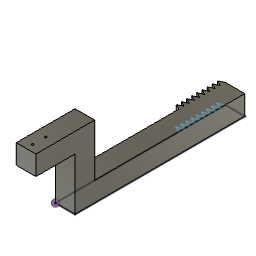
ClaspRight v1 (Autodesk Fusion 360 design; units mm, degrees)
Autodesk Fusion 360 part; units mm, degrees
sketch "Sketch1" plane through (0, 0, 0) normal (0, 0, 1) x (1, 0, 0)
  line L0 (0, 0) -> (19.05, 0)
  line L1 (19.05, 0) -> (19.05, 165.1)
  line L2 (19.05, 165.1) -> (0, 165.1)
  line L3 (0, 165.1) -> (0, 0)
  line L4 (0, 165.1) -> (-5, 162.5)
  line L5 (-5, 162.5) -> (0, 160)
  line L6 (-5, 157.5) -> (0, 160)
  line L7 (-5, 157.5) -> (0, 155)
  line L8 (0, 155) -> (-5, 152.5)
  line L9 (-5, 152.5) -> (0, 150)
  line L10 (0, 150) -> (-5, 147.5)
  line L11 (-5, 147.5) -> (0, 145)
  line L12 (0, 145) -> (-5, 142.5)
  line L13 (-5, 142.5) -> (0, 140)
  line L14 (0, 140) -> (-5, 137.5)
  line L15 (-5, 137.5) -> (0, 135)
  line L16 (0, 135) -> (-5, 132.5)
  line L17 (-5, 132.5) -> (0, 130)
  line L18 (0, 130) -> (-5, 127.5)
  line L19 (-5, 127.5) -> (0, 125)
  line L20 (0, 125) -> (-5, 122.5)
  line L21 (-5, 122.5) -> (0, 120)
  dimension "d2" = 19.05
  dimension "d3" = 165.1
  constraint horizontal L0
  constraint vertical L1
  constraint horizontal L2
  constraint vertical L3
  constraint coincident L0.start L3.end
  constraint coincident L3 L5.end
  constraint coincident L3 L7.end
  constraint parallel L5 L7
  constraint parallel L6 L8
  constraint coincident L3 L9.end
  constraint parallel L7 L9
  constraint parallel L8 L10
  constraint coincident L3 L11.end
  constraint parallel L9 L11
  constraint parallel L10 L12
  constraint coincident L3 L13.end
  constraint parallel L11 L13
  constraint parallel L12 L14
  constraint coincident L3 L15.end
  constraint parallel L13 L15
  constraint parallel L14 L16
  constraint coincident L3 L17.end
  constraint parallel L15 L17
  constraint parallel L16 L18
  constraint coincident L3 L19.end
  constraint parallel L17 L19
  constraint parallel L18 L20
  constraint coincident L3 L21.end
  constraint parallel L19 L21
  measures "d2" distance of L1.end L2.end
  measures "d3" distance of L0.end L1.end
extrude "Extrude1" add sketch "Sketch1" along normal blind 19.05 contours L0 L1 L2 L3 | L3 L20 L21 | L3 L18 L19 | L3 L16 L17 | L3 L14 L15 | L3 L8 L9 | L3 L12 L13 | L3 L10 L11
sketch "Sketch2" plane through (0, 0, 19.05) normal (0, 0, 1) x (-1, 0, 0)
  line L0 (5, -122.5) -> (0, -120)
  line L1 (0, -120) -> (0, 0)
  line L2 (0, 0) -> (-19.05, 0)
  line L3 (-19.05, 0) -> (-19.05, -165.1)
  line L4 (-19.05, -165.1) -> (0, -165.1)
  line L5 (0, -165.1) -> (0, -155)
  line L6 (0, -155) -> (5, -152.5)
  line L7 (5, -152.5) -> (0, -150)
  line L8 (0, -150) -> (5, -147.5)
  line L9 (5, -147.5) -> (0, -145)
  line L10 (0, -145) -> (5, -142.5)
  line L11 (5, -142.5) -> (0, -140)
  line L12 (0, -140) -> (5, -137.5)
  line L13 (5, -137.5) -> (0, -135)
  line L14 (0, -135) -> (5, -132.5)
  line L15 (5, -132.5) -> (0, -130)
  line L16 (0, -130) -> (5, -127.5)
  line L17 (5, -127.5) -> (0, -125)
  line L18 (0, -125) -> (5, -122.5)
  line L19 (0, 0) -> (-19.05, 0)
  line L20 (-19.05, 0) -> (-19.05, -19.05)
  line L21 (-19.05, -19.05) -> (0, -19.05)
  line L22 (0, -19.05) -> (0, 0)
  dimension "d6" = 19.05
  dimension "d7" = 19.05
  constraint horizontal L19
  constraint vertical L20
  constraint horizontal L21
  constraint vertical L22
  constraint coincident L3 L20.end
  constraint coincident L1.end L2.start
  measures "d6" distance of L20.end L21.end
  measures "d7" distance of L1.end L21.end
extrude "Extrude2" add sketch "Sketch2" along normal blind 50.8 contours L1 L2 L3 L19 L20 L21 L22
sketch "Sketch3" plane through (0, 0, 0) normal (0, -1, 0) x (1, 0, 0)
  line L0 (0, 0) -> (19.05, 0)
  line L1 (19.05, 0) -> (19.05, 69.85)
  line L2 (19.05, 69.85) -> (0, 69.85)
  line L3 (0, 69.85) -> (0, 0)
  line L4 (0, 69.85) -> (19.05, 69.85)
  line L5 (19.05, 69.85) -> (19.05, 50.8)
  line L6 (19.05, 50.8) -> (0, 50.8)
  line L7 (0, 50.8) -> (0, 69.85)
  dimension "d10" = 19.05
  constraint horizontal L4
  constraint vertical L5
  constraint horizontal L6
  constraint vertical L7
  constraint coincident L1 L5.end
  constraint coincident L2.end L3.start
  measures "d10" distance of L2.end L6.end
extrude "Extrude3" add sketch "Sketch3" along normal blind 38.1 contours L1 L2 L3 L4 L5 L6 L7
extrude "Extrude4" add sketch "Sketch1" along normal blind 19.05 contours L3 L4 L5 | L3 L6 L7
sketch "Sketch4" plane through (0, 0, 69.85) normal (0, 0, 1) x (-1, 0, 0)
  line L0 (0, -19.05) -> (0, 38.1)
  line L1 (0, 38.1) -> (-19.05, 38.1)
  line L2 (-19.05, 38.1) -> (-19.05, -19.05)
  line L3 (-19.05, -19.05) -> (0, -19.05)
  circle A0 centre (-9.525, 19.05) radius 1
  circle A1 centre (-9.525, 31.75) radius 1.0988
  dimension "d15" = 12.7
  dimension "d16" = 9.525
  dimension "d17" = 6.35
  measures "d15" distance of A0.centre A1.centre
  measures "d16" distance of L2 A1.centre
  measures "d17" distance of L1 A1.centre
extrude "Extrude5" cut sketch "Sketch4" against normal blind 33 contours A0 | A1
